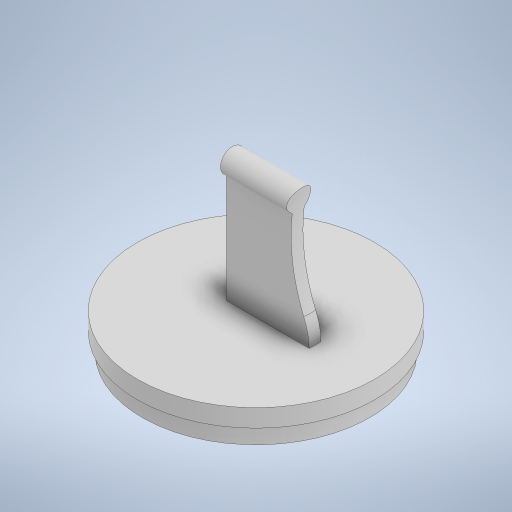
# Autodesk Inventor part: Basic seal circle head beserk simple a
Saved by Autodesk Inventor 2024 (Build 280153000, 153)
## iProperties
Created: 2023-05-18
Part Number: Basic seal circle head beserk simple a
Material: Generic
Document SubType Name: Modeling
Designer: newic
Density: 1 g/cm^3
Appearance: Default
Author: newic
Autodesk Inventor part; units mm, degrees
(part 1 of 2)
ref_plane "YZ Plane" through (0, 0, 0) normal (1, 0, 0) x (0, 1, 0)
ref_plane "XZ Plane" through (0, 0, 0) normal (0, 1, 0) x (-1, 0, 0)
ref_plane "XY Plane" through (0, 0, 0) normal (0, 0, 1) x (1, 0, 0)
sketch "Sketch1" plane through (0, 0, 0) normal (0, 1, 0) x (-1, 0, 0)
  circle A0 centre (0, 0) radius 12.7
  line L0 (12.7, 12.7) -> (12.7, -12.7) construction
  line L1 (12.7, -12.7) -> (-12.7, -12.7) construction
  line L2 (-12.7, -12.7) -> (-12.7, 12.7) construction
  line L3 (-12.7, 12.7) -> (12.7, 12.7) construction
  circle A1 centre (0, 0) radius 12.1875
  circle A2 centre (0, 0) radius 11.5722
  line L4 (12.7, 0) -> (-28.224, 0)
  spline S0 degree 4 poles (7.5608, 0) (7.5871, -0.2498) (7.5716, -0.8639) (7.6635, -1.72) (7.771, -2.5827) (7.8796, -3.1444) (8.0283, -3.9996) (8.2528, -4.7367) (8.3389, -5.0369) (8.4927, -5.4299) (8.607, -5.7477) (8.7077, -5.9466) (8.7297, -6.0528) (8.7259, -6.1323) (8.6915, -6.2267) (8.6084, -6.3073) (8.4656, -6.4322) (8.3108, -6.5585) (7.9581, -6.8561) (7.7627, -7.0404) (7.5994, -7.1572) (7.2874, -7.4352) (7.0492, -7.6385) (6.8557, -7.7767) (6.6363, -7.9955) (6.5444, -8.04) (6.425, -8.09) (6.3049, -8.0852) (6.1612, -8.0439) (5.8673, -7.9243) (5.2047, -7.7184) (4.9544, -7.6282) (4.5834, -7.5418) (3.9869, -7.3825) (3.5585, -7.2836) (3.3261, -7.2353) (2.6639, -7.1283) (2.4923, -7.0851) (1.885, -7.0109) (1.2249, -6.9515) (0.9978, -6.9092) (-0.0967, -6.8274) (-0.0908, -6.8879) (-0.9888, -6.8956) (-1.4498, -6.994) (-2.157, -7.03) (-2.8755, -7.1861) (-3.3866, -7.2397) (-4.3934, -7.4794) (-4.8139, -7.612) (-5.3152, -7.7313) (-5.615, -7.8484) (-5.8655, -7.9444) (-6.1746, -8.0443) (-6.2691, -8.0783) (-6.3955, -8.0918) (-6.486, -8.0779) (-6.6705, -8.0058) (-6.661, -7.9168) (-6.8879, -7.7874) (-7.0089, -7.6489) (-7.1824, -7.5178) (-7.3229, -7.3873) (-7.5822, -7.175) (-7.7931, -7.0025) (-8.0826, -6.7466) (-8.2527, -6.613) (-8.4352, -6.4317) (-8.5724, -6.3549) (-8.667, -6.2237) (-8.6858, -6.2037) (-8.7162, -6.092) (-8.7131, -6.0317) (-8.695, -5.9554) (-8.5854, -5.7043) (-8.4697, -5.4626) (-8.3913, -5.2076) (-8.2879, -4.9538) (-8.1958, -4.6121) (-8.0468, -4.045) (-7.9725, -3.8304) (-7.7592, -2.661) (-7.6907, -2.1909) (-7.6151, -1.4373) (-7.564, -0.619) (-7.5516, -0.3428) (-7.5554, -0.0046) (-7.5638, 0) knots 0 0 0 0 0 0.039296 0.055908 0.073069 0.090127 0.10618 0.121509 0.134965 0.146316 0.15619 0.164179 0.170591 0.176443 0.182863 0.190407 0.199969 0.210544 0.221389 0.232964 0.244031 0.25516 0.266564 0.276442 0.284967 0.292352 0.298886 0.30652 0.31685 0.32851 0.341463 0.355682 0.368855 0.381917 0.395666 0.408085 0.420945 0.435034 0.448763 0.464427 0.47884 0.493305 0.508372 0.522986 0.539358 0.555691 0.57306 0.589942 0.605994 0.620829 0.633477 0.645128 0.655027 0.663676 0.671144 0.677933 0.684628 0.692084 0.700281 0.708721 0.71788 0.727519 0.737693 0.74871 0.760009 0.770972 0.781161 0.789961 0.797299 0.803676 0.809144 0.814179 0.820577 0.828361 0.837524 0.847989 0.859019 0.870721 0.882901 0.897625 0.913523 0.930287 0.948149 0.964022 0.978288 1 1 1 1 1
  spline S1 degree 4 poles (7.5608, 0) (7.5871, 0.2498) (7.5716, 0.8639) (7.6635, 1.72) (7.771, 2.5827) (7.8796, 3.1444) (8.0283, 3.9996) (8.2528, 4.7367) (8.3389, 5.0368) (8.4927, 5.4299) (8.607, 5.7477) (8.7077, 5.9466) (8.7297, 6.0528) (8.7259, 6.1323) (8.6915, 6.2267) (8.6084, 6.3073) (8.4656, 6.4322) (8.3108, 6.5585) (7.9581, 6.8561) (7.7627, 7.0404) (7.5994, 7.1572) (7.2874, 7.4352) (7.0492, 7.6385) (6.8557, 7.7767) (6.6363, 7.9955) (6.5444, 8.04) (6.425, 8.09) (6.3049, 8.0852) (6.1612, 8.0439) (5.8673, 7.9243) (5.2047, 7.7184) (4.9544, 7.6282) (4.5834, 7.5418) (3.9869, 7.3825) (3.5585, 7.2836) (3.3261, 7.2353) (2.6639, 7.1283) (2.4923, 7.0851) (1.885, 7.0109) (1.2249, 6.9515) (0.9978, 6.9092) (-0.0967, 6.8274) (-0.0908, 6.8879) (-0.9888, 6.8956) (-1.4498, 6.994) (-2.157, 7.03) (-2.8755, 7.1861) (-3.3866, 7.2397) (-4.3934, 7.4794) (-4.8139, 7.612) (-5.3152, 7.7313) (-5.615, 7.8484) (-5.8655, 7.9444) (-6.1746, 8.0443) (-6.2691, 8.0783) (-6.3955, 8.0918) (-6.486, 8.0779) (-6.6705, 8.0058) (-6.661, 7.9168) (-6.8879, 7.7874) (-7.0089, 7.6489) (-7.1824, 7.5178) (-7.3229, 7.3873) (-7.5822, 7.175) (-7.7931, 7.0025) (-8.0826, 6.7466) (-8.2527, 6.613) (-8.4352, 6.4317) (-8.5724, 6.3549) (-8.667, 6.2237) (-8.6858, 6.2037) (-8.7162, 6.092) (-8.7131, 6.0317) (-8.695, 5.9554) (-8.5854, 5.7043) (-8.4697, 5.4626) (-8.3913, 5.2076) (-8.2879, 4.9538) (-8.1958, 4.6121) (-8.0468, 4.045) (-7.9725, 3.8304) (-7.7592, 2.661) (-7.6907, 2.1909) (-7.6151, 1.4373) (-7.564, 0.619) (-7.5516, 0.3428) (-7.5554, 0.0046) (-7.5638, 0) knots 0 0 0 0 0 0.039296 0.055908 0.073069 0.090127 0.10618 0.121509 0.134965 0.146316 0.15619 0.164179 0.170591 0.176443 0.182863 0.190407 0.199969 0.210544 0.221389 0.232964 0.244031 0.25516 0.266564 0.276442 0.284967 0.292352 0.298886 0.30652 0.31685 0.32851 0.341463 0.355682 0.368855 0.381917 0.395666 0.408085 0.420945 0.435034 0.448763 0.464427 0.47884 0.493305 0.508372 0.522986 0.539358 0.555691 0.57306 0.589942 0.605994 0.620829 0.633477 0.645128 0.655027 0.663676 0.671144 0.677933 0.684628 0.692084 0.700281 0.708721 0.71788 0.727519 0.737693 0.74871 0.760009 0.770972 0.781161 0.789961 0.797299 0.803676 0.809144 0.814179 0.820577 0.828361 0.837524 0.847989 0.859019 0.870721 0.882901 0.897625 0.913523 0.930287 0.948149 0.964022 0.978288 1 1 1 1 1
  spline S2 degree 4 poles (6.6698, 0) (6.6871, -0.3978) (6.6713, -0.7815) (6.7409, -1.5229) (6.8536, -2.5936) (6.9252, -2.906) (7.0997, -3.8444) (7.2267, -4.3825) (7.3633, -4.7956) (7.4896, -5.3512) (7.6112, -5.5391) (7.6677, -5.7689) (7.6975, -5.7897) (7.7062, -5.8965) (7.6285, -5.9815) (7.572, -6.0514) (7.3996, -6.178) (7.1331, -6.4178) (6.9588, -6.5681) (6.6364, -6.8323) (6.5004, -6.9541) (6.3704, -7.0647) (6.3037, -7.1086) (6.2234, -7.1388) (6.1631, -7.1283) (6.0268, -7.0924) (5.9076, -7.0514) (5.5806, -6.952) (5.3855, -6.8908) (5.038, -6.812) (4.9484, -6.7624) (4.2814, -6.6028) (4.0156, -6.5429) (3.8882, -6.5183) (3.3037, -6.3965) (2.8824, -6.3286) (2.5502, -6.2731) (2.4025, -6.2241) (1.6246, -6.1518) (1.37, -6.0874) (1.1134, -6.1) (0.6072, -6.0267) (0.5913, -6.054) (0.1833, -6.0225) (0.0815, -6.0123) (-0.2846, -6.0335) (-0.5883, -6.0362) (-0.9225, -6.0806) (-1.3996, -6.1121) (-1.6329, -6.1378) (-2.1126, -6.197) (-2.4639, -6.2503) (-2.782, -6.3007) (-3.1586, -6.3702) (-3.2077, -6.3787) (-3.7538, -6.4818) (-4.0918, -6.5436) (-4.3482, -6.6242) (-4.8814, -6.7303) (-5.2054, -6.8556) (-5.5087, -6.9063) (-5.6572, -6.9822) (-5.9526, -7.0706) (-6.1139, -7.1317) (-6.1762, -7.1269) (-6.2789, -7.1205) (-6.425, -7.0257) (-6.5484, -6.9167) (-6.706, -6.7703) (-6.9687, -6.5457) (-7.0919, -6.4669) (-7.3885, -6.1958) (-7.4865, -6.1263) (-7.6283, -5.9822) (-7.6822, -5.9316) (-7.7081, -5.8596) (-7.7006, -5.7637) (-7.6112, -5.6344) (-7.5282, -5.3549) (-7.4652, -5.1836) (-7.3295, -4.7829) (-7.1819, -4.1547) (-7.1117, -3.848) (-6.9524, -3.2013) (-6.8781, -2.6524) (-6.8463, -2.4403) (-6.7659, -1.8396) (-6.735, -1.4493) (-6.7089, -1.1731) (-6.6784, -0.6337) (-6.6716, -0.3941) (-6.6731, -0.0474) (-6.6763, 0) knots 0 0 0 0 0 0.039448 0.055349 0.072269 0.088737 0.104506 0.120552 0.134467 0.146293 0.155548 0.162505 0.168442 0.174025 0.180717 0.189099 0.198791 0.210185 0.221737 0.232089 0.240921 0.247815 0.253612 0.259204 0.265359 0.273108 0.282299 0.292472 0.302955 0.314654 0.326295 0.337305 0.349803 0.361846 0.37389 0.386284 0.399242 0.411449 0.423896 0.437159 0.44785 0.458402 0.468238 0.477683 0.488335 0.499312 0.51153 0.523717 0.536339 0.54908 0.561517 0.573881 0.584661 0.595665 0.606838 0.61814 0.631344 0.644301 0.656608 0.668396 0.679342 0.688982 0.697238 0.704622 0.711137 0.717919 0.725945 0.735426 0.745345 0.756153 0.766663 0.776344 0.78489 0.791619 0.7976 0.803458 0.810655 0.819014 0.829148 0.841433 0.854403 0.869138 0.884301 0.898105 0.912368 0.925751 0.938316 0.951323 0.9634 0.975086 1 1 1 1 1
  spline S3 degree 4 poles (6.6698, 0) (6.6871, 0.3978) (6.6713, 0.7814) (6.7409, 1.5229) (6.8536, 2.5936) (6.9252, 2.906) (7.0997, 3.8444) (7.2267, 4.3825) (7.3633, 4.7956) (7.4896, 5.3512) (7.6112, 5.5391) (7.6677, 5.7689) (7.6975, 5.7897) (7.7062, 5.8965) (7.6285, 5.9815) (7.572, 6.0514) (7.3996, 6.178) (7.1331, 6.4178) (6.9588, 6.5681) (6.6364, 6.8323) (6.5004, 6.9541) (6.3704, 7.0646) (6.3037, 7.1085) (6.2234, 7.1388) (6.1631, 7.1283) (6.0268, 7.0924) (5.9076, 7.0514) (5.5806, 6.952) (5.3855, 6.8908) (5.038, 6.812) (4.9484, 6.7624) (4.2814, 6.6028) (4.0156, 6.5429) (3.8882, 6.5183) (3.3037, 6.3965) (2.8824, 6.3286) (2.5502, 6.2731) (2.4025, 6.2241) (1.6246, 6.1517) (1.37, 6.0874) (1.1134, 6.1) (0.6072, 6.0267) (0.5913, 6.054) (0.1833, 6.0225) (0.0815, 6.0123) (-0.2846, 6.0335) (-0.5883, 6.0362) (-0.9225, 6.0806) (-1.3996, 6.1121) (-1.6329, 6.1378) (-2.1126, 6.197) (-2.4639, 6.2503) (-2.782, 6.3007) (-3.1586, 6.3702) (-3.2077, 6.3787) (-3.7538, 6.4818) (-4.0918, 6.5436) (-4.3482, 6.6242) (-4.8814, 6.7303) (-5.2054, 6.8556) (-5.5087, 6.9063) (-5.6572, 6.9822) (-5.9526, 7.0706) (-6.1139, 7.1317) (-6.1762, 7.1269) (-6.2789, 7.1205) (-6.425, 7.0257) (-6.5484, 6.9166) (-6.706, 6.7703) (-6.9687, 6.5457) (-7.0919, 6.4669) (-7.3885, 6.1958) (-7.4865, 6.1263) (-7.6283, 5.9822) (-7.6822, 5.9316) (-7.7081, 5.8596) (-7.7006, 5.7637) (-7.6112, 5.6344) (-7.5282, 5.3549) (-7.4652, 5.1836) (-7.3295, 4.7829) (-7.1819, 4.1547) (-7.1117, 3.848) (-6.9524, 3.2013) (-6.8781, 2.6524) (-6.8463, 2.4403) (-6.7659, 1.8396) (-6.735, 1.4493) (-6.7089, 1.1731) (-6.6784, 0.6337) (-6.6716, 0.3941) (-6.6731, 0.0474) (-6.6763, 0) knots 0 0 0 0 0 0.039448 0.055349 0.072269 0.088737 0.104506 0.120552 0.134467 0.146293 0.155548 0.162505 0.168442 0.174025 0.180717 0.189099 0.198791 0.210185 0.221737 0.232089 0.240921 0.247815 0.253612 0.259204 0.265359 0.273108 0.282299 0.292472 0.302955 0.314654 0.326295 0.337305 0.349803 0.361846 0.37389 0.386284 0.399242 0.411449 0.423896 0.437159 0.44785 0.458402 0.468238 0.477683 0.488335 0.499312 0.51153 0.523717 0.536339 0.54908 0.561517 0.573881 0.584661 0.595665 0.606838 0.61814 0.631344 0.644301 0.656608 0.668396 0.679342 0.688982 0.697238 0.704622 0.711137 0.717919 0.725945 0.735426 0.745345 0.756153 0.766663 0.776344 0.78489 0.791619 0.7976 0.803458 0.810655 0.819014 0.829148 0.841433 0.854403 0.869138 0.884301 0.898105 0.912368 0.925751 0.938316 0.951323 0.9634 0.975086 1 1 1 1 1
  line L5 (1.0941, 0) -> (1.0941, -2.0952)
  line L6 (1.0941, -2.0952) -> (3.9049, -2.2474)
  line L7 (3.9049, -2.2474) -> (4.7904, -1.5612)
  line L8 (-0.5884, 0) -> (-0.5898, -1.9938)
  line L9 (-0.5898, -1.9938) -> (-4.3298, -1.7894)
  line L10 (-4.3298, -1.7894) -> (-5.2324, -1.0809)
  line L11 (5.0927, -1.7005) -> (5.1051, -4.9152)
  line L12 (4.7853, -5.0014) -> (3.8243, -3.9243)
  line L13 (3.8243, -3.9243) -> (-4.2884, -3.485)
  line L14 (-4.2884, -3.485) -> (-5.2324, -4.5455)
  line L15 (-5.5377, -4.4469) -> (-5.5322, -1.2345)
  arc A3 (5.0927, -1.7005) -> (4.7904, -1.5612) centre (4.931, -1.6537) ccw
  arc A4 (4.7853, -5.0014) -> (5.1051, -4.9152) centre (4.9338, -4.9158) ccw
  arc A5 (-5.5377, -4.4469) -> (-5.2324, -4.5455) centre (-5.3693, -4.4472) ccw
  arc A6 (-5.2324, -1.0809) -> (-5.5322, -1.2345) centre (-5.368, -1.1857) ccw
  line L16 (1.0941, 0) -> (1.0941, 2.0952)
  line L17 (1.0941, 2.0952) -> (3.9049, 2.2474)
  line L18 (3.9049, 2.2474) -> (4.7904, 1.5612)
  line L19 (-0.5884, 0) -> (-0.5898, 1.9938)
  line L20 (-0.5898, 1.9938) -> (-4.3298, 1.7894)
  line L21 (-4.3298, 1.7894) -> (-5.2324, 1.0809)
  line L22 (5.0927, 1.7005) -> (5.1051, 4.9152)
  line L23 (4.7853, 5.0014) -> (3.8243, 3.9243)
  line L24 (3.8243, 3.9243) -> (-4.2884, 3.485)
  line L25 (-4.2884, 3.485) -> (-5.2324, 4.5455)
  arc A7 (4.7904, 1.5612) -> (5.0927, 1.7005) centre (4.931, 1.6537) ccw
  arc A8 (5.1051, 4.9152) -> (4.7853, 5.0014) centre (4.9338, 4.9158) ccw
  arc A9 (-5.2324, 4.5455) -> (-5.5377, 4.4469) centre (-5.3693, 4.4472) ccw
  arc A10 (-5.5322, 1.2345) -> (-5.2324, 1.0809) centre (-5.368, 1.1857) ccw
  line L26 (-5.5377, 4.4469) -> (-5.5322, 1.2345)
  point P0 (7.582, -0.4475)
  point P1 (7.6181, -1.1897)
  point P2 (7.6938, -1.9478)
  point P3 (7.7753, -2.5562)
  point P4 (7.8781, -3.1491)
  point P5 (8.0672, -4.0731)
  point P6 (8.2624, -4.7725)
  point P7 (8.3673, -5.0974)
  point P8 (8.5065, -5.4722)
  point P9 (8.6396, -5.8063)
  point P10 (8.7107, -5.9813)
  point P11 (8.7259, -6.0648)
  point P12 (8.7208, -6.1314)
  point P13 (8.6916, -6.2086)
  point P14 (8.625, -6.2893)
  point P15 (8.5035, -6.398)
  point P16 (8.3259, -6.5472)
  point P17 (7.9666, -6.8536)
  point P18 (7.7597, -7.0347)
  point P19 (7.5972, -7.1666)
  point P20 (7.2997, -7.4223)
  point P21 (7.0358, -7.6431)
  point P22 (6.8133, -7.8257)
  point P23 (6.615, -7.9971)
  point P24 (6.5232, -8.0478)
  point P25 (6.4269, -8.0794)
  point P26 (6.3307, -8.0824)
  point P27 (6.2157, -8.0568)
  point P28 (5.939, -7.9581)
  point P29 (5.2485, -7.7291)
  point P30 (4.9341, -7.6303)
  point P31 (4.5863, -7.5395)
  point P32 (3.9767, -7.3836)
  point P33 (3.5714, -7.2881)
  point P34 (3.2721, -7.2292)
  point P35 (2.7391, -7.1371)
  point P36 (2.4628, -7.0879)
  point P37 (1.9303, -7.0199)
  point P38 (1.3001, -6.9537)
  point P39 (0.8618, -6.905)
  point P40 (0.0288, -6.8555)
  point P41 (-0.2052, -6.8728)
  point P42 (-0.8545, -6.91)
  point P43 (-1.4645, -6.978)
  point P44 (-2.1388, -7.0515)
  point P45 (-2.824, -7.1641)
  point P46 (-3.4525, -7.2709)
  point P47 (-4.4053, -7.4924)
  point P48 (-4.9149, -7.6324)
  point P49 (-5.3455, -7.7526)
  point P50 (-5.6379, -7.8568)
  point P51 (-5.9277, -7.9626)
  point P52 (-6.1933, -8.0512)
  point P53 (-6.2931, -8.0776)
  point P54 (-6.3884, -8.0863)
  point P55 (-6.4903, -8.0706)
  point P56 (-6.6308, -8.0034)
  point P57 (-6.6877, -7.9317)
  point P58 (-6.8516, -7.7973)
  point P59 (-7.0164, -7.6529)
  point P60 (-7.1659, -7.5263)
  point P61 (-7.3162, -7.3971)
  point P62 (-7.5527, -7.1992)
  point P63 (-7.8063, -6.9879)
  point P64 (-8.0883, -6.7461)
  point P65 (-8.2789, -6.5822)
  point P66 (-8.4597, -6.4263)
  point P67 (-8.5958, -6.3127)
  point P68 (-8.6662, -6.2262)
  point P69 (-8.6877, -6.1869)
  point P70 (-8.71, -6.101)
  point P71 (-8.7118, -6.043)
  point P72 (-8.6987, -5.9829)
  point P73 (-8.6117, -5.7675)
  point P74 (-8.4802, -5.4672)
  point P75 (-8.3902, -5.2184)
  point P76 (-8.3037, -4.977)
  point P77 (-8.2036, -4.6385)
  point P78 (-8.0738, -4.1578)
  point P79 (-7.9798, -3.7988)
  point P80 (-7.7876, -2.7953)
  point P81 (-7.688, -2.1188)
  point P82 (-7.614, -1.3524)
  point P83 (-7.5689, -0.6701)
  point P84 (-7.5559, -0.2905)
  point P85 (-7.5591, -0.0322)
  point P86 (7.582, 0.4475)
  point P87 (7.6181, 1.1897)
  point P88 (7.6938, 1.9478)
  point P89 (7.7753, 2.5562)
  point P90 (7.8781, 3.1491)
  point P91 (8.0672, 4.0731)
  point P92 (8.2624, 4.7725)
  point P93 (8.3673, 5.0973)
  point P94 (8.5065, 5.4722)
  point P95 (8.6396, 5.8063)
  point P96 (8.7107, 5.9813)
  point P97 (8.7259, 6.0648)
  point P98 (8.7208, 6.1314)
  point P99 (8.6916, 6.2085)
  point P100 (8.625, 6.2893)
  point P101 (8.5035, 6.398)
  point P102 (8.3259, 6.5472)
  point P103 (7.9666, 6.8536)
  point P104 (7.7597, 7.0347)
  point P105 (7.5972, 7.1666)
  point P106 (7.2997, 7.4223)
  point P107 (7.0358, 7.6431)
  point P108 (6.8133, 7.8257)
  point P109 (6.615, 7.997)
  point P110 (6.5232, 8.0478)
  point P111 (6.4269, 8.0794)
  point P112 (6.3307, 8.0824)
  point P113 (6.2157, 8.0568)
  point P114 (5.939, 7.9581)
  point P115 (5.2485, 7.7291)
  point P116 (4.9341, 7.6303)
  point P117 (4.5863, 7.5395)
  point P118 (3.9767, 7.3836)
  point P119 (3.5714, 7.2881)
  point P120 (3.2721, 7.2292)
  point P121 (2.7391, 7.1371)
  point P122 (2.4628, 7.0879)
  point P123 (1.9303, 7.0199)
  point P124 (1.3001, 6.9537)
  point P125 (0.8618, 6.905)
  point P126 (0.0288, 6.8555)
  point P127 (-0.2052, 6.8727)
  point P128 (-0.8545, 6.91)
  point P129 (-1.4645, 6.978)
  point P130 (-2.1388, 7.0515)
  point P131 (-2.824, 7.1641)
  point P132 (-3.4525, 7.2709)
  point P133 (-4.4053, 7.4924)
  point P134 (-4.9149, 7.6324)
  point P135 (-5.3455, 7.7526)
  point P136 (-5.6379, 7.8568)
  point P137 (-5.9277, 7.9626)
  point P138 (-6.1933, 8.0512)
  point P139 (-6.2931, 8.0776)
  point P140 (-6.3884, 8.0863)
  point P141 (-6.4903, 8.0706)
  point P142 (-6.6308, 8.0034)
  point P143 (-6.6877, 7.9317)
  point P144 (-6.8516, 7.7973)
  point P145 (-7.0164, 7.6529)
  point P146 (-7.1659, 7.5263)
  point P147 (-7.3162, 7.3971)
  point P148 (-7.5527, 7.1992)
  point P149 (-7.8063, 6.9879)
  point P150 (-8.0883, 6.746)
  point P151 (-8.2789, 6.5822)
  point P152 (-8.4597, 6.4263)
  point P153 (-8.5958, 6.3127)
  point P154 (-8.6662, 6.2262)
  point P155 (-8.6877, 6.1869)
  point P156 (-8.71, 6.101)
  point P157 (-8.7118, 6.043)
  point P158 (-8.6987, 5.9829)
  point P159 (-8.6117, 5.7675)
  point P160 (-8.4802, 5.4672)
  point P161 (-8.3902, 5.2183)
  point P162 (-8.3037, 4.977)
  point P163 (-8.2036, 4.6385)
  point P164 (-8.0738, 4.1578)
  point P165 (-7.9798, 3.7987)
  point P166 (-7.7876, 2.7953)
  point P167 (-7.688, 2.1188)
  point P168 (-7.614, 1.3524)
  point P169 (-7.5689, 0.6701)
  point P170 (-7.5559, 0.2905)
  point P171 (-7.5591, 0.0322)
  point P172 (6.6836, -0.5412)
  point P173 (6.7072, -1.0761)
  point P174 (6.774, -1.8261)
  point P175 (6.8568, -2.5341)
  point P176 (6.9346, -2.9728)
  point P177 (7.1026, -3.8229)
  point P178 (7.2446, -4.4136)
  point P179 (7.3804, -4.8955)
  point P180 (7.5322, -5.3935)
  point P181 (7.6322, -5.6381)
  point P182 (7.6779, -5.7675)
  point P183 (7.6936, -5.8064)
  point P184 (7.6937, -5.8803)
  point P185 (7.6435, -5.9655)
  point P186 (7.5821, -6.0322)
  point P187 (7.446, -6.1471)
  point P188 (7.1705, -6.3831)
  point P189 (6.9233, -6.5957)
  point P190 (6.6151, -6.8536)
  point P191 (6.4599, -6.9878)
  point P192 (6.3548, -7.0726)
  point P193 (6.2905, -7.111)
  point P194 (6.2287, -7.1307)
  point P195 (6.1718, -7.1283)
  point P196 (6.068, -7.1023)
  point P197 (5.9271, -7.0591)
  point P198 (5.6207, -6.9639)
  point P199 (5.36, -6.8886)
  dimension "d0" = 25.4
  dimension "d32" = 25.4
  dimension "d39" = 25.4
  constraints: 195 symmetric about line, 46 end point, 17 point on circle, 11 centre point, 6 point on line, 3 coincident, 2 tangent, 1 horizontal, 1 midpoint, 1 perpendicular, 368 other
  measures "d0" diameter of A0
  measures "d32" distance of L2.end L0.start
  measures "d39" distance of L0.start L0.end
extrude "Extrusion1" add sketch "Sketch1" along normal blind 1.905 contours L4 A2 A1 | A1 L4 A2 | S0 L4 S2 | L4 S3 S1 | L5 L6 L7 A3 L11 A4 L12 L13 L14 A5 L15 A6 L10 L9 L8 L4 | L4 L19 L20 L21 A10 L26 A9 L25 L24 L23 A8 L22 A7 L18 L17 L16
sketch "Sketch2" plane through (0, 1.905, 0) normal (0, 1, 0) x (1, 0, 0)
  line L0 (12.7067, 12.7) -> (12.7067, -12.7) construction
  line L1 (12.7067, -12.7) -> (-12.6933, -12.7) construction
  line L2 (-12.6933, -12.7) -> (-12.6933, 12.7) construction
  line L3 (-12.6933, 12.7) -> (12.7067, 12.7) construction
  circle A0 centre (0, 0) radius 12.1875 projected
  line L4 (-12.1875, 0) -> (-18.0724, 0)
  circle A1 centre (0, 0) radius 12.7
  dimension "d92" = 25.4
  dimension "d98" = 25.4
  constraints: 2 end point, 1 centre point, 1 coincident, 1 horizontal, 1 horizontal alignment, 3 other
  measures "d92" distance of L2.end L0.start
  measures "d98" diameter of A1
extrude "Extrusion2" add sketch "Sketch2" along normal blind 1.905 contours A0 | A1
sketch "Sketch3" plane through (0, 0, 0) normal (0, 0, 1) x (1, 0, 0)
  line L0 (0, 0) -> (0, 88.9)
  line L1 (134.3126, 257.1223) -> (473.4262, 257.1223) construction
  line L2 (473.4262, 257.1223) -> (473.4262, 17.1036) construction
  line L3 (473.4262, 17.1036) -> (134.3126, 17.1036) construction
  line L4 (134.3126, 17.1036) -> (134.3126, 257.1223) construction
  circle A0 centre (112.6944, 39.6279) radius 12.7
  circle A1 centre (0, 44.45) radius 5.08
  circle A2 centre (0, 77.1578) radius 10.16
  line L5 (0, 44.45) -> (0, 3.81)
  line L6 (12.7, 3.81) -> (-12.7, 3.81) projected
  circle A3 centre (0, 24.13) radius 5.08
  circle A4 centre (5.0788, 24.2425) radius 2.54
  circle A5 centre (-4.9792, 23.1233) radius 2.54
  line L7 (-4.9792, 23.1233) -> (-13.9595, 32.1035)
  line L8 (-4.9792, 23.1233) -> (7.7208, 23.1233) construction
  line L9 (5.0788, 24.2425) -> (14.059, 33.2227)
  line L10 (5.0788, 24.2425) -> (17.7788, 24.2425) construction
  line L11 (5.0788, 24.2425) -> (12.9329, 19.8885)
  line L12 (-4.9792, 23.1233) -> (-13.9595, 14.143)
  line L13 (-4.9792, 23.1233) -> (7.7208, 23.1233) construction
  arc A6 (9.9682, 75.1929) -> (6.8748, 26.0385) centre (108.777, 44.3001) ccw
  arc A7 (-6.7753, 24.9193) -> (-9.9499, 75.1021) centre (-109.0911, 43.6386) ccw
  circle A8 centre (0, 3.81) radius 6.35
  line L14 (0, 24.13) -> (0, 3.81)
  circle A9 centre (0, 13.97) radius 4.445
  arc A10 (-6.35, 3.81) -> (-6.7753, 21.3272) centre (-23.0464, 12.1684) ccw
  arc A11 (7.3002, 23.011) -> (5.779, 6.4416) centre (22.4276, 13.2676) ccw
  point P0 (0, 87.3178)
  point P1 (0, 3.81)
  point P2 (6.35, 3.81)
  dimension "d101" = 88.9
  dimension "d103" = 25.4
  dimension "d118" = 10.16
  dimension "d122" = 20.32
  dimension "d123" = 10.16
  dimension "d124" = 5.08
  dimension "d125" = 5.08
  dimension "d126" = 12.7
  dimension "d127" = 135
  dimension "d128" = 12.7
  dimension "d129" = 45
  dimension "d130" = 12.7
  dimension "d131" = 135
  dimension "d132" = 12.7
  dimension "d133" = 8.89
  constraints: 20 end point, 18 point on circle, 12 centre point, 6 point on line, 4 midpoint, 3 equal length, 3 horizontal, 3 tangent, 1 coincident, 1 collinear, 1 vertical, 2 other
  measures "d101" distance of L0.start L0.end
  measures "d103" diameter of A0
  measures "d118" diameter of A1
  measures "d122" diameter of A2
  measures "d123" diameter of A3
  measures "d124" diameter of A4
  measures "d125" diameter of A5
  measures "d126" distance of L7.start L7.end
  measures "d127" angle of L8 L7
  measures "d128" distance of L9.start L9.end
  measures "d129" angle of L10 L9
  measures "d130" distance of L7.start L12.end
  measures "d131" angle of L12 L13
  measures "d132" diameter of A8
  measures "d133" diameter of A9
revolve "Revolution1" add sketch "Sketch3" angle 360 about axis through (0, 44.45, 0) along (0, -1, 0) picked at (0.2042, 9.7508) picked at (0.3297, 15.6262) picked at (3.3442, 44.0732) contours L0 A9 A8 L6 | L0 A8 A9 | L0 A9 A8 | A9 A11 A8 | L0 A3 A4 A11 A9 | L0 A3 A4 | A4 A3 L11 A11 | A4 A3 | L11 L9 A4 | L0 A1 A2 A6 A4 A3 | A4 L9 A3 | L0 A1 | A2 L0 A6
sketch "Sketch4" plane through (0, 0, 0) normal (1, 0, 0) x (0, 1, 0)
  line L0 (3.81, 6.35) -> (3.81, -6.35) projected
  line L1 (3.81, 0) -> (16.51, 0)
  line L2 (16.51, 0) -> (16.51, -0.635)
  line L3 (16.51, -0.635) -> (3.81, -0.635)
  line L4 (3.81, -0.635) -> (3.81, 0.635)
  line L5 (3.81, 0.635) -> (16.51, 0.635)
  line L6 (16.51, 0.635) -> (16.51, -0.635)
  circle A0 centre (16.51, 0) radius 1.27
  line L7 (3.81, -0.635) -> (3.81, -16.3637)
  line L8 (3.81, 0.635) -> (3.81, 15.8696)
  line L9 (3.81, 15.8696) -> (99.2843, 27.0509)
  line L10 (99.2843, 27.0509) -> (97.7935, -45.0686)
  line L11 (97.7935, -45.0686) -> (3.81, -16.3637)
  point P0 (15.4101, 0.635)
  point P1 (15.4101, -0.635)
  dimension "d140" = 12.7
  dimension "d141" = 0.635
  dimension "d142" = 12.7
  dimension "d143" = 1.27
  dimension "d144" = 2.54
  constraints: 22 end point, 2 horizontal, 2 parallel, 2 perpendicular, 1 centre point, 1 coincident, 1 midpoint, 1 point on line, 1 vertical
  measures "d140" distance of L1.start L1.end
  measures "d141" distance of L1.end L2.end
  measures "d142" distance of L4.end L5.end
  measures "d143" distance of L3.end L4.end
  measures "d144" diameter of A0
extrude "Extrusion3" cut sketch "Sketch4" along normal mid plane 25.4 contours L8 L9 L10 L11 L7 L0 L3 A0 L5
sketch "Sketch5" plane through (0, 0, 0) normal (0, 0, 1) x (1, 0, 0)
  line L0 (5.009, 17.78) -> (-5.009, 17.78) projected
  line L1 (0, 17.78) -> (-2.54, 17.78)
  line L2 (12.7, 3.81) -> (-12.7, 3.81) projected
  line L3 (-2.54, 17.78) -> (-12.7, 17.78)
  line L4 (-12.7, 17.78) -> (-12.7, 3.81)
  line L5 (-12.7, 3.81) -> (-2.54, 3.81)
  line L6 (-2.54, 3.81) -> (-2.54, 17.78)
  point P0 (0, 0)
  dimension "d147" = 2.54
  constraints: 10 end point, 2 parallel, 1 horizontal, 1 midpoint, 1 perpendicular, 1 point on line
  measures "d147" distance of L1.start L1.end
extrude "Extrusion4" cut sketch "Sketch5" along normal mid plane 25.4
sketch "Sketch6" plane through (0, 0, 0) normal (0, -1, 0) x (1, 0, 0)
  circle A0 centre (0, 0) radius 11.5722
  constraints: 1 centre point, 1 coincident
extrude "Extrusion5" cut sketch "Sketch6" against normal blind 1.905
sketch "Sketch7" plane through (0, 1.905, 0) normal (0, -1, 0) x (1, 0, 0)
  line L0 (14.6102, 14.5451) -> (14.6102, -14.7607) construction
  line L1 (14.6102, -14.7607) -> (-14.6956, -14.7607) construction
  line L2 (-14.6956, -14.7607) -> (-14.6956, 14.5451) construction
  line L3 (-14.6956, 14.5451) -> (14.6102, 14.5451) construction
  arc A0 (-7.2117, 6.6079) -> (-4.2178, 9.2498) centre (-13.2655, 16.4856) ccw
  circle A1 centre (0, 0) radius 11.5722 projected
  line L4 (11.5722, 0) -> (-11.5722, 0)
  arc A2 (-6.5517, 5.8618) -> (-7.2117, 6.6079) centre (-8.749, 4.583) ccw
  arc A3 (-6.5517, 5.8618) -> (-8.4692, 3.1505) centre (-0.144, -0.7036) ccw
  arc A4 (-10.4266, 0) -> (-8.4692, 3.1505) centre (-12.0826, 3.2122) ccw
  arc A5 (3.6422, 8.0666) -> (2.7975, 7.2546) centre (4.0073, 6.8415) ccw
  arc A6 (3.8192, 7.977) -> (4.0431, 7.3031) centre (5.9598, 8.3141) ccw
  arc A7 (5.3195, 8.3498) -> (4.1892, 7.2546) centre (7.8749, 4.5817) ccw
  arc A8 (6.3873, 8.274) -> (5.3195, 8.3498) centre (5.8229, 7.8826) ccw
  arc A9 (7.1115, 7.3995) -> (6.3873, 8.274) centre (3.473, 5.1233) ccw
  arc A10 (7.1115, 7.3995) -> (8.8095, 5.4013) centre (14.7867, 12.2009) ccw
  arc A11 (8.8159, 4.7146) -> (8.8095, 5.4013) centre (8.0641, 5.051) ccw
  arc A12 (8.8159, 4.7146) -> (7.5857, 0.8693) centre (17.5205, -0.1896) ccw
  arc A13 (7.4873, 0.7361) -> (6.6954, 0) centre (7.9897, -0.5986) ccw
  arc A14 (-4.2178, 9.2498) -> (3.4467, 5.8404) centre (6.4252, 22.8564) ccw
  arc A15 (3.8192, 7.977) -> (3.6422, 8.0666) centre (3.6924, 7.9461) ccw
  arc A16 (2.7975, 7.2546) -> (2.8198, 7.014) centre (3.1484, 7.1658) ccw
  arc A17 (2.8198, 7.014) -> (3.6134, 6.1469) centre (4.7537, 7.9871) ccw
  arc A18 (3.7326, 5.8942) -> (3.6134, 6.1469) centre (3.5815, 5.9774) ccw
  arc A19 (3.4467, 5.8404) -> (3.7326, 5.8942) centre (3.555, 6.0517) ccw
  arc A20 (4.0431, 7.3031) -> (4.1892, 7.2546) centre (4.126, 7.3086) ccw
  arc A21 (7.4873, 0.7361) -> (7.5857, 0.8693) centre (7.3838, 0.9154) ccw
  arc A22 (7.2212, 1.0369) -> (6.3496, 0.16) centre (7.9897, -0.5986) ccw
  arc A23 (8.4739, 4.8838) -> (7.2212, 1.0369) centre (17.5205, -0.1896) ccw
  arc A24 (8.4739, 4.8838) -> (8.4884, 5.1768) centre (8.0641, 5.051) ccw
  arc A25 (6.7885, 7.1974) -> (8.4884, 5.1768) centre (14.7867, 12.2009) ccw
  arc A26 (6.7885, 7.1974) -> (6.0922, 8.0275) centre (3.473, 5.1233) ccw
  arc A27 (6.0922, 8.0275) -> (5.5987, 8.0906) centre (5.8229, 7.8826) ccw
  arc A28 (5.5333, 8.0345) -> (4.4924, 7.0238) centre (7.8749, 4.5817) ccw
  arc A29 (3.6831, 7.1701) -> (4.4924, 7.0238) centre (4.126, 7.3086) ccw
  arc A30 (3.5161, 7.5925) -> (3.6831, 7.1701) centre (5.9598, 8.3141) ccw
  arc A31 (3.5161, 7.5925) -> (3.1704, 7.1653) centre (4.0073, 6.8415) ccw
  arc A32 (3.1704, 7.1653) -> (3.7741, 6.4962) centre (4.7537, 7.9871) ccw
  arc A33 (4.0433, 5.6724) -> (3.7741, 6.4962) centre (3.5815, 5.9774) ccw
  arc A34 (3.3375, 5.4728) -> (4.0433, 5.6724) centre (3.555, 6.0517) ccw
  arc A35 (-4.1578, 8.7241) -> (3.3375, 5.4728) centre (6.4252, 22.8564) ccw
  arc A36 (-6.5903, 6.5542) -> (-4.1578, 8.7241) centre (-13.2655, 16.4856) ccw
  arc A37 (-6.0825, 5.7812) -> (-6.5903, 6.5542) centre (-8.749, 4.583) ccw
  arc A38 (-6.0825, 5.7812) -> (-8.0906, 3.0607) centre (-0.144, -0.7036) ccw
  arc A39 (-9.7075, 0) -> (-8.0906, 3.0607) centre (-12.0826, 3.2122) ccw
  line L5 (5.5333, 8.0345) -> (5.5987, 8.0906)
  arc A40 (6.3496, 0.16) -> (6.2968, 0) centre (6.8009, -0.0778) ccw
  arc A41 (-8.5913, 0) -> (-7.4478, 2.5301) centre (-11.3121, 2.753) ccw
  arc A42 (-5.6429, 5.2004) -> (-7.4363, 2.5761) centre (1.2908, -1.4629) ccw
  arc A43 (-5.608, 6.2854) -> (-5.6086, 5.3051) centre (-1.9398, 5.7931) ccw
  arc A44 (-5.5548, 6.3727) -> (-4.291, 7.5795) centre (-8.8335, 11.0711) ccw
  arc A45 (-4.1175, 7.6062) -> (2.2722, 4.7981) centre (6.1174, 22.222) ccw
  arc A46 (2.2722, 4.7981) -> (4.2214, 4.7477) centre (3.4297, 11.8425) ccw
  arc A47 (4.724, 5.2467) -> (4.3171, 4.81) centre (5.4844, 4.1301) ccw
  line L6 (4.7788, 5.3385) -> (4.865, 6.1688)
  arc A48 (5.6142, 7.0713) -> (4.8748, 6.2062) centre (6.652, 5.4357) ccw
  arc A49 (5.7851, 7.0385) -> (7.4394, 5.0423) centre (21.9288, 18.7334) ccw
  arc A50 (7.4994, 4.6966) -> (6.5516, 1.5843) centre (20.1293, -0.8502) ccw
  arc A51 (6.4883, 1.4695) -> (5.7632, 0.6705) centre (10.7854, -3.1592) ccw
  arc A52 (5.7027, 0.5315) -> (5.676, 0) centre (7.9095, 0.1543) ccw
  arc A53 (5.3478, 0.7031) -> (5.2943, 0) centre (7.9095, 0.1543) ccw
  arc A54 (6.1151, 1.6403) -> (5.4031, 0.8255) centre (10.7854, -3.1592) ccw
  arc A55 (7.0534, 4.6234) -> (6.2056, 1.8083) centre (20.1293, -0.8502) ccw
  arc A56 (5.7144, 6.4934) -> (6.994, 4.9612) centre (21.9288, 18.7334) ccw
  arc A57 (5.5207, 6.5041) -> (5.2494, 6.1094) centre (6.652, 5.4357) ccw
  line L7 (5.2375, 6.0675) -> (5.1378, 5.1067)
  arc A58 (5.0662, 5.0052) -> (4.5785, 4.4765) centre (5.4844, 4.1301) ccw
  arc A59 (2.2105, 4.4222) -> (4.4775, 4.396) centre (3.4297, 11.8425) ccw
  arc A60 (-4.0461, 7.0951) -> (2.1901, 4.4261) centre (6.1174, 22.222) ccw
  arc A61 (-5.1975, 6.1604) -> (-4.2129, 7.0728) centre (-8.8335, 11.0711) ccw
  arc A62 (-5.2484, 6.0689) -> (-5.2032, 5.1821) centre (-1.9398, 5.7931) ccw
  arc A63 (-5.2383, 5.0689) -> (-7.0605, 2.4804) centre (1.2908, -1.4629) ccw
  arc A64 (-8.0721, 0) -> (-7.0723, 2.4357) centre (-11.3121, 2.753) ccw
  line L8 (2.1901, 4.4261) -> (2.2105, 4.4222)
  arc A65 (6.4883, 1.4695) -> (6.5516, 1.5843) centre (6.3182, 1.6379) ccw
  arc A66 (7.4994, 4.6966) -> (7.4394, 5.0423) centre (7.2087, 4.8242) ccw
  arc A67 (7.0534, 4.6234) -> (6.994, 4.9612) centre (6.7606, 4.7459) ccw
  arc A68 (6.1151, 1.6403) -> (6.2056, 1.8083) centre (5.8937, 1.8679) ccw
  arc A69 (5.4031, 0.8255) -> (5.3478, 0.7031) centre (5.6583, 0.6366) ccw
  arc A70 (5.7632, 0.6705) -> (5.7027, 0.5315) centre (6.0157, 0.478) ccw
  arc A71 (5.7144, 6.4934) -> (5.5207, 6.5041) centre (5.6131, 6.4169) ccw
  arc A72 (5.7851, 7.0385) -> (5.6142, 7.0713) centre (5.6823, 6.964) ccw
  arc A73 (4.8748, 6.2062) -> (4.865, 6.1688) centre (4.9913, 6.1557) ccw
  arc A74 (5.2494, 6.1094) -> (5.2375, 6.0675) centre (5.3639, 6.0544) ccw
  arc A75 (5.0662, 5.0052) -> (5.1378, 5.1067) centre (5.0115, 5.1198) ccw
  arc A76 (4.724, 5.2467) -> (4.7788, 5.3385) centre (4.6525, 5.3516) ccw
  arc A77 (4.2214, 4.7477) -> (4.3171, 4.81) centre (4.2073, 4.8739) ccw
  arc A78 (4.4775, 4.396) -> (4.5785, 4.4765) centre (4.4598, 4.5218) ccw
  arc A79 (-4.0461, 7.0951) -> (-4.2129, 7.0728) centre (-4.1169, 6.9897) ccw
  arc A80 (-4.1175, 7.6062) -> (-4.291, 7.5795) centre (-4.1904, 7.5021) ccw
  arc A81 (-5.5548, 6.3727) -> (-5.608, 6.2854) centre (-5.4822, 6.2685) ccw
  arc A82 (-5.1975, 6.1604) -> (-5.2484, 6.0689) centre (-5.1219, 6.0583) ccw
  arc A83 (-5.2383, 5.0689) -> (-5.2032, 5.1821) centre (-5.3281, 5.1587) ccw
  arc A84 (-5.6429, 5.2004) -> (-5.6086, 5.3051) centre (-5.7345, 5.2884) ccw
  arc A85 (-7.4363, 2.5761) -> (-7.4478, 2.5301) centre (-7.321, 2.5228) ccw
  arc A86 (-7.0605, 2.4804) -> (-7.0723, 2.4357) centre (-6.9456, 2.4262) ccw
  line L9 (-0.3479, 0) -> (-0.3479, 1.9307)
  line L10 (-0.5384, 2.1212) -> (-3.2789, 2.1212)
  line L11 (-3.4694, 1.9307) -> (-3.4694, 1.2225)
  line L12 (-3.5329, 1.159) -> (-3.8795, 1.159)
  line L13 (-3.943, 1.2225) -> (-3.943, 4.3325)
  line L14 (-3.8795, 4.396) -> (-3.5329, 4.396)
  line L15 (-3.4694, 4.3325) -> (-3.4694, 3.4264)
  line L16 (-3.2809, 3.2359) -> (2.8648, 3.1705)
  line L17 (3.0574, 3.359) -> (3.0631, 3.8994)
  line L18 (3.1273, 3.9622) -> (3.5187, 3.958)
  line L19 (3.5815, 3.8945) -> (3.5815, 1.0412)
  line L20 (3.518, 0.9777) -> (3.1273, 0.9777)
  line L21 (3.0638, 1.0412) -> (3.0638, 1.9307)
  line L22 (2.8733, 2.1212) -> (0.3391, 2.1212)
  line L23 (0.1486, 1.9327) -> (0.128, 0)
  arc A87 (0.3391, 2.1212) -> (0.1486, 1.9327) centre (0.3391, 1.9307) ccw
  arc A88 (-0.3479, 1.9307) -> (-0.5384, 2.1212) centre (-0.5384, 1.9307) ccw
  arc A89 (-3.2789, 2.1212) -> (-3.4694, 1.9307) centre (-3.2789, 1.9307) ccw
  arc A90 (-3.4694, 3.4264) -> (-3.2809, 3.2359) centre (-3.2789, 3.4264) ccw
  arc A91 (2.8648, 3.1705) -> (3.0574, 3.359) centre (2.8669, 3.361) ccw
  arc A92 (3.0638, 1.9307) -> (2.8733, 2.1212) centre (2.8733, 1.9307) ccw
  arc A93 (3.0638, 1.0412) -> (3.1273, 0.9777) centre (3.1273, 1.0412) ccw
  arc A94 (3.518, 0.9777) -> (3.5815, 1.0412) centre (3.518, 1.0412) ccw
  arc A95 (3.5815, 3.8945) -> (3.5187, 3.958) centre (3.518, 3.8945) ccw
  arc A96 (3.1273, 3.9622) -> (3.0631, 3.8994) centre (3.1266, 3.8987) ccw
  arc A97 (-3.4694, 4.3325) -> (-3.5329, 4.396) centre (-3.5329, 4.3325) ccw
  arc A98 (-3.8795, 4.396) -> (-3.943, 4.3325) centre (-3.8795, 4.3325) ccw
  arc A99 (-3.943, 1.2225) -> (-3.8795, 1.159) centre (-3.8795, 1.2225) ccw
  arc A100 (-3.5329, 1.159) -> (-3.4694, 1.2225) centre (-3.5329, 1.2225) ccw
  arc A101 (-4.2178, -9.2498) -> (-7.2117, -6.6079) centre (-13.2655, -16.4856) ccw
  circle A102 centre (0, 0) radius 11.5722
  arc A103 (-7.2117, -6.6079) -> (-6.5517, -5.8618) centre (-8.749, -4.583) ccw
  arc A104 (-8.4692, -3.1505) -> (-6.5517, -5.8618) centre (-0.144, 0.7036) ccw
  arc A105 (-8.4692, -3.1505) -> (-10.4266, 0) centre (-12.0826, -3.2122) ccw
  arc A106 (2.7975, -7.2546) -> (3.6422, -8.0666) centre (4.0073, -6.8415) ccw
  arc A107 (4.0431, -7.3031) -> (3.8192, -7.977) centre (5.9598, -8.3141) ccw
  arc A108 (4.1892, -7.2546) -> (5.3195, -8.3498) centre (7.8749, -4.5817) ccw
  arc A109 (5.3195, -8.3498) -> (6.3873, -8.274) centre (5.8229, -7.8826) ccw
  arc A110 (6.3873, -8.274) -> (7.1115, -7.3995) centre (3.473, -5.1233) ccw
  arc A111 (8.8095, -5.4013) -> (7.1115, -7.3995) centre (14.7867, -12.2009) ccw
  arc A112 (8.8095, -5.4013) -> (8.8159, -4.7146) centre (8.0641, -5.051) ccw
  arc A113 (7.5857, -0.8693) -> (8.8159, -4.7146) centre (17.5205, 0.1896) ccw
  arc A114 (6.6954, 0) -> (7.4873, -0.7361) centre (7.9897, 0.5986) ccw
  arc A115 (3.4467, -5.8404) -> (-4.2178, -9.2498) centre (6.4252, -22.8564) ccw
  arc A116 (3.6422, -8.0666) -> (3.8192, -7.977) centre (3.6924, -7.9461) ccw
  arc A117 (2.8198, -7.014) -> (2.7975, -7.2546) centre (3.1484, -7.1658) ccw
  arc A118 (3.6134, -6.1469) -> (2.8198, -7.014) centre (4.7537, -7.9871) ccw
  arc A119 (3.6134, -6.1469) -> (3.7326, -5.8942) centre (3.5815, -5.9774) ccw
  arc A120 (3.7326, -5.8942) -> (3.4467, -5.8404) centre (3.555, -6.0517) ccw
  arc A121 (4.1892, -7.2546) -> (4.0431, -7.3031) centre (4.126, -7.3086) ccw
  arc A122 (7.5857, -0.8693) -> (7.4873, -0.7361) centre (7.3838, -0.9154) ccw
  arc A123 (6.3496, -0.16) -> (7.2212, -1.0369) centre (7.9897, 0.5986) ccw
  arc A124 (7.2212, -1.0369) -> (8.4739, -4.8838) centre (17.5205, 0.1896) ccw
  arc A125 (8.4884, -5.1768) -> (8.4739, -4.8838) centre (8.0641, -5.051) ccw
  arc A126 (8.4884, -5.1768) -> (6.7885, -7.1974) centre (14.7867, -12.2009) ccw
  arc A127 (6.0922, -8.0275) -> (6.7885, -7.1974) centre (3.473, -5.1233) ccw
  arc A128 (5.5987, -8.0906) -> (6.0922, -8.0275) centre (5.8229, -7.8826) ccw
  arc A129 (4.4924, -7.0238) -> (5.5333, -8.0345) centre (7.8749, -4.5817) ccw
  arc A130 (4.4924, -7.0238) -> (3.6831, -7.1701) centre (4.126, -7.3086) ccw
  arc A131 (3.6831, -7.1701) -> (3.5161, -7.5925) centre (5.9598, -8.3141) ccw
  arc A132 (3.1704, -7.1653) -> (3.5161, -7.5925) centre (4.0073, -6.8415) ccw
  arc A133 (3.7741, -6.4962) -> (3.1704, -7.1653) centre (4.7537, -7.9871) ccw
  arc A134 (3.7741, -6.4962) -> (4.0433, -5.6724) centre (3.5815, -5.9774) ccw
  arc A135 (4.0433, -5.6724) -> (3.3375, -5.4728) centre (3.555, -6.0517) ccw
  arc A136 (3.3375, -5.4728) -> (-4.1578, -8.7241) centre (6.4252, -22.8564) ccw
  arc A137 (-4.1578, -8.7241) -> (-6.5903, -6.5542) centre (-13.2655, -16.4856) ccw
  arc A138 (-6.5903, -6.5542) -> (-6.0825, -5.7812) centre (-8.749, -4.583) ccw
  arc A139 (-8.0906, -3.0607) -> (-6.0825, -5.7812) centre (-0.144, 0.7036) ccw
  arc A140 (-8.0906, -3.0607) -> (-9.7075, 0) centre (-12.0826, -3.2122) ccw
  line L24 (5.5333, -8.0345) -> (5.5987, -8.0906)
  arc A141 (6.2968, 0) -> (6.3496, -0.16) centre (6.8009, 0.0778) ccw
  arc A142 (-7.4478, -2.5301) -> (-8.5913, 0) centre (-11.3121, -2.753) ccw
  arc A143 (-7.4363, -2.5761) -> (-5.6429, -5.2004) centre (1.2908, 1.4629) ccw
  arc A144 (-5.6086, -5.3051) -> (-5.608, -6.2854) centre (-1.9398, -5.7931) ccw
  arc A145 (-4.291, -7.5795) -> (-5.5548, -6.3727) centre (-8.8335, -11.0711) ccw
  arc A146 (2.2722, -4.7981) -> (-4.1175, -7.6062) centre (6.1174, -22.222) ccw
  arc A147 (4.2214, -4.7477) -> (2.2722, -4.7981) centre (3.4297, -11.8425) ccw
  arc A148 (4.3171, -4.81) -> (4.724, -5.2467) centre (5.4844, -4.1301) ccw
  line L25 (4.7788, -5.3385) -> (4.865, -6.1688)
  arc A149 (4.8748, -6.2062) -> (5.6142, -7.0713) centre (6.652, -5.4357) ccw
  arc A150 (7.4394, -5.0423) -> (5.7851, -7.0385) centre (21.9288, -18.7334) ccw
  arc A151 (6.5516, -1.5843) -> (7.4994, -4.6966) centre (20.1293, 0.8502) ccw
  arc A152 (5.7632, -0.6705) -> (6.4883, -1.4695) centre (10.7854, 3.1592) ccw
  arc A153 (5.676, 0) -> (5.7027, -0.5315) centre (7.9095, -0.1543) ccw
  arc A154 (5.2943, 0) -> (5.3478, -0.7031) centre (7.9095, -0.1543) ccw
  arc A155 (5.4031, -0.8255) -> (6.1151, -1.6403) centre (10.7854, 3.1592) ccw
  arc A156 (6.2056, -1.8083) -> (7.0534, -4.6234) centre (20.1293, 0.8502) ccw
  arc A157 (6.994, -4.9612) -> (5.7144, -6.4934) centre (21.9288, -18.7334) ccw
  arc A158 (5.2494, -6.1094) -> (5.5207, -6.5041) centre (6.652, -5.4357) ccw
  line L26 (5.2375, -6.0675) -> (5.1378, -5.1067)
  arc A159 (4.5785, -4.4765) -> (5.0662, -5.0052) centre (5.4844, -4.1301) ccw
  arc A160 (4.4775, -4.396) -> (2.2105, -4.4222) centre (3.4297, -11.8425) ccw
  arc A161 (2.1901, -4.4261) -> (-4.0461, -7.0951) centre (6.1174, -22.222) ccw
  arc A162 (-4.2129, -7.0728) -> (-5.1975, -6.1604) centre (-8.8335, -11.0711) ccw
  arc A163 (-5.2032, -5.1821) -> (-5.2484, -6.0689) centre (-1.9398, -5.7931) ccw
  arc A164 (-7.0605, -2.4804) -> (-5.2383, -5.0689) centre (1.2908, 1.4629) ccw
  arc A165 (-7.0723, -2.4357) -> (-8.0721, 0) centre (-11.3121, -2.753) ccw
  line L27 (2.1901, -4.4261) -> (2.2105, -4.4222)
  arc A166 (6.5516, -1.5843) -> (6.4883, -1.4695) centre (6.3182, -1.6379) ccw
  arc A167 (7.4394, -5.0423) -> (7.4994, -4.6966) centre (7.2087, -4.8242) ccw
  arc A168 (6.994, -4.9612) -> (7.0534, -4.6234) centre (6.7606, -4.7459) ccw
  arc A169 (6.2056, -1.8083) -> (6.1151, -1.6403) centre (5.8937, -1.8679) ccw
  arc A170 (5.3478, -0.7031) -> (5.4031, -0.8255) centre (5.6583, -0.6366) ccw
  arc A171 (5.7027, -0.5315) -> (5.7632, -0.6705) centre (6.0157, -0.478) ccw
  arc A172 (5.5207, -6.5041) -> (5.7144, -6.4934) centre (5.6131, -6.4169) ccw
  arc A173 (5.6142, -7.0713) -> (5.7851, -7.0385) centre (5.6823, -6.964) ccw
  arc A174 (4.865, -6.1688) -> (4.8748, -6.2062) centre (4.9913, -6.1557) ccw
  arc A175 (5.2375, -6.0675) -> (5.2494, -6.1094) centre (5.3639, -6.0544) ccw
  arc A176 (5.1378, -5.1067) -> (5.0662, -5.0052) centre (5.0115, -5.1198) ccw
  arc A177 (4.7788, -5.3385) -> (4.724, -5.2467) centre (4.6525, -5.3516) ccw
  arc A178 (4.3171, -4.81) -> (4.2214, -4.7477) centre (4.2073, -4.8739) ccw
  arc A179 (4.5785, -4.4765) -> (4.4775, -4.396) centre (4.4598, -4.5218) ccw
  arc A180 (-4.2129, -7.0728) -> (-4.0461, -7.0951) centre (-4.1169, -6.9897) ccw
  arc A181 (-4.291, -7.5795) -> (-4.1175, -7.6062) centre (-4.1904, -7.5021) ccw
  arc A182 (-5.608, -6.2854) -> (-5.5548, -6.3727) centre (-5.4822, -6.2685) ccw
  arc A183 (-5.2484, -6.0689) -> (-5.1975, -6.1604) centre (-5.1219, -6.0583) ccw
  arc A184 (-5.2032, -5.1821) -> (-5.2383, -5.0689) centre (-5.3281, -5.1587) ccw
  arc A185 (-5.6086, -5.3051) -> (-5.6429, -5.2004) centre (-5.7345, -5.2884) ccw
  arc A186 (-7.4478, -2.5301) -> (-7.4363, -2.5761) centre (-7.321, -2.5228) ccw
  arc A187 (-7.0723, -2.4357) -> (-7.0605, -2.4804) centre (-6.9456, -2.4262) ccw
  line L28 (-0.3479, 0) -> (-0.3479, -1.9307)
  line L29 (-0.5384, -2.1212) -> (-3.2789, -2.1212)
  line L30 (-3.4694, -1.9307) -> (-3.4694, -1.2225)
  line L31 (-3.5329, -1.159) -> (-3.8795, -1.159)
  line L32 (-3.943, -1.2225) -> (-3.943, -4.3325)
  line L33 (-3.8795, -4.396) -> (-3.5329, -4.396)
  line L34 (-3.4694, -4.3325) -> (-3.4694, -3.4264)
  line L35 (-3.2809, -3.2359) -> (2.8648, -3.1705)
  line L36 (3.0574, -3.359) -> (3.0631, -3.8994)
  line L37 (3.1273, -3.9622) -> (3.5187, -3.958)
  line L38 (3.5815, -3.8945) -> (3.5815, -1.0412)
  line L39 (3.518, -0.9777) -> (3.1273, -0.9777)
  line L40 (3.0638, -1.0412) -> (3.0638, -1.9307)
  line L41 (2.8733, -2.1212) -> (0.3391, -2.1212)
  line L42 (0.1486, -1.9327) -> (0.128, 0)
  arc A188 (0.1486, -1.9327) -> (0.3391, -2.1212) centre (0.3391, -1.9307) ccw
  arc A189 (-0.5384, -2.1212) -> (-0.3479, -1.9307) centre (-0.5384, -1.9307) ccw
  arc A190 (-3.4694, -1.9307) -> (-3.2789, -2.1212) centre (-3.2789, -1.9307) ccw
  arc A191 (-3.2809, -3.2359) -> (-3.4694, -3.4264) centre (-3.2789, -3.4264) ccw
  arc A192 (3.0574, -3.359) -> (2.8648, -3.1705) centre (2.8669, -3.361) ccw
  arc A193 (2.8733, -2.1212) -> (3.0638, -1.9307) centre (2.8733, -1.9307) ccw
  arc A194 (3.1273, -0.9777) -> (3.0638, -1.0412) centre (3.1273, -1.0412) ccw
  arc A195 (3.5815, -1.0412) -> (3.518, -0.9777) centre (3.518, -1.0412) ccw
  arc A196 (3.5187, -3.958) -> (3.5815, -3.8945) centre (3.518, -3.8945) ccw
  arc A197 (3.0631, -3.8994) -> (3.1273, -3.9622) centre (3.1266, -3.8987) ccw
  arc A198 (-3.5329, -4.396) -> (-3.4694, -4.3325) centre (-3.5329, -4.3325) ccw
  arc A199 (-3.943, -4.3325) -> (-3.8795, -4.396) centre (-3.8795, -4.3325) ccw
  arc A200 (-3.8795, -1.159) -> (-3.943, -1.2225) centre (-3.8795, -1.2225) ccw
  arc A201 (-3.4694, -1.2225) -> (-3.5329, -1.159) centre (-3.5329, -1.2225) ccw
  point P0 (4.7726, 5.2782)
  point P1 (4.867, 6.1879)
  point P2 (5.2398, 6.089)
  point P3 (5.1301, 5.033)
  point P4 (-3.4694, 4.396)
  point P5 (-3.4694, 3.2379)
  point P6 (3.0638, 2.1212)
  point P7 (0.1506, 2.1212)
  point P8 (4.7726, -5.2782)
  point P9 (4.867, -6.1879)
  point P10 (5.2398, -6.089)
  point P11 (5.1301, -5.033)
  point P12 (-3.4694, -4.396)
  point P13 (-3.4694, -3.2379)
  point P14 (3.0638, -2.1212)
  point P15 (0.1506, -2.1212)
  point P16 (5.3195, 8.3498)
  point P17 (-8.4692, 3.1505)
  dimension "d195" = 0.381
  dimension "d196" = 0.381
  dimension "d197" = 0.381
  dimension "d198" = 0.381
  dimension "d201" = 0.381
  dimension "d202" = 0.381
  dimension "d203" = 0.3175
  dimension "d204" = 0.127
  dimension "d208" = 0.1905
  dimension "d209" = 0.0635
  constraints: 416 point on circle, 201 centre point, 197 vertical alignment, 131 equal radius, 76 end point, 70 tangent, 32 point on line, 10 perpendicular, 1 concentric, 1 parallel, 1 vertical, 33 other
  measures "d195" radial gap between concentric circles of A12 A23
  measures "d196" radial gap between concentric circles of A7 A28
  measures "d197" radial gap between concentric circles of A14 A35
  measures "d198" radial gap between concentric circles of A4 A39
  measures "d201" radial gap between concentric circles of A52 A53
  measures "d202" radial gap between concentric circles of A45 A60
  measures "d203" radius of A66
  measures "d204" radius of A71
  measures "d208" radius of A87
  measures "d209" radius of A93
extrude "Extrusion6" add sketch "Sketch7" along normal blind 1.905 contours A0 A14 A19 A18 A17 A16 A5 A15 A6 A20 A7 A8 A9 A10 A11 A12 A21 A13 L4 A40 A22 A23 A24 A25 A26 A27 L5 A28 A29 A30 A31 A32 A33 A34 A35 A36 A37 A38 A39 A4 A3 A2 | L4 A140 A139 A138 A137 A136 A135 A134 A133 A132 A131 A130 A129 L24 A128 A127 A126 A125 A124 A123 A141 A114 A122 A113 A112 A111 A110 A109 A108 A121 A107 A116 A106 A117 A118 A119 A120 A115 A101 A103 A104 A105 | A41 A85 A42 A84 A43 A81 A44 A80 A45 A46 A77 A47 A76 L6 A73 A48 A72 A49 A66 A50 A65 A51 A70 A52 L4 A53 A69 A54 A68 A55 A67 A56 A71 A57 A74 L7 A75 A58 A78 A59 L8 A60 A79 A61 A82 A62 A83 A63 A86 A64 | L4 A165 A187 A164 A184 A163 A183 A162 A180 A161 L27 A160 A179 A159 A176 L26 A175 A158 A172 A157 A168 A156 A169 A155 A170 A154 A153 A171 A152 A166 A151 A167 A150 A173 A149 A174 L25 A177 A148 A178 A147 A146 A181 A145 A182 A144 A185 A143 A186 A142 | L9 A88 L10 A89 L11 A100 L12 A99 L13 A98 L14 A97 L15 A90 L16 A91 L17 A96 L18 A95 L19 A94 L20 A93 L21 A92 L22 A87 L23 L4 | L4 L42 A188 L41 A193 L40 A194 L39 A195 L38 A196 L37 A197 L36 A192 L35 A191 L34 A198 L33 A199 L32 A200 L31 A201 L30 A190 L29 A189 L28
sketch "Sketch8" plane through (0, 0, 0) normal (0, -1, 0) x (1, 0, 0)
  circle A0 centre (0, 0) radius 11.5722
  constraints: 1 centre point, 1 coincident
extrude "Extrusion7" cut sketch "Sketch8" against normal blind 1.905